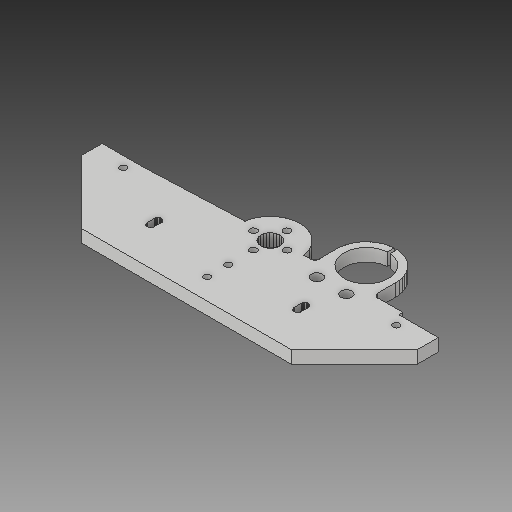
# Autodesk Inventor part: Rear-Bed-Holder-Lower
Saved by Autodesk Inventor 2017 (Build 210142000, 142)
## iProperties
Created: 2016-07-12
Part Number: Rear-Bed-Holder-Lower
Material: Generic
Document SubType Name: Modeling
Designer: joshmamo
Density: 1 g/cm^3
Appearance: Default
Author: joshmamo
Autodesk Inventor part; units mm, degrees
ref_plane "YZ Plane" through (0, 0, 0) normal (1, 0, 0) x (0, 1, 0)
ref_plane "XZ Plane" through (0, 0, 0) normal (0, 1, 0) x (-1, 0, 0)
ref_plane "XY Plane" through (0, 0, 0) normal (0, 0, 1) x (1, 0, 0)
sketch "Sketch1" plane through (0, 0, 0) normal (0, 1, 0) x (-1, 0, 0)
  line L0 (324.9839, 293.9621) -> (323.9081, 293.4902)
  line L1 (323.9081, 293.4902) -> (322.9911, 292.756)
  line L2 (322.9911, 292.756) -> (322.2953, 291.8095)
  line L3 (322.2953, 291.8095) -> (321.8683, 290.7151)
  line L4 (321.8683, 290.7151) -> (321.739, 289.5475)
  line L5 (321.739, 289.5475) -> (321.9163, 288.3862)
  line L6 (321.9163, 288.3862) -> (322.3882, 287.3104)
  line L7 (322.3882, 287.3104) -> (323.1224, 286.3934)
  line L8 (323.1224, 286.3934) -> (324.0689, 285.6977)
  line L9 (324.0689, 285.6977) -> (325.1633, 285.2706)
  line L10 (325.1633, 285.2706) -> (326.3309, 285.1413)
  line L11 (326.3309, 285.1413) -> (327.4922, 285.3187)
  line L12 (327.4922, 285.3187) -> (328.568, 285.7905)
  line L13 (328.568, 285.7905) -> (329.485, 286.5247)
  line L14 (329.485, 286.5247) -> (330.1807, 287.4713)
  line L15 (330.1807, 287.4713) -> (330.6078, 288.5656)
  line L16 (330.6078, 288.5656) -> (330.7371, 289.7332)
  line L17 (330.7371, 289.7332) -> (330.5598, 290.8945)
  line L18 (330.5598, 290.8945) -> (330.0879, 291.9703)
  line L19 (330.0879, 291.9703) -> (329.3537, 292.8873)
  line L20 (329.3537, 292.8873) -> (328.4072, 293.5831)
  line L21 (328.4072, 293.5831) -> (327.3128, 294.0101)
  line L22 (327.3128, 294.0101) -> (326.1452, 294.1394)
  line L23 (326.1452, 294.1394) -> (324.9839, 293.9621)
  line L24 (362.7103, 307.2904) -> (362.8801, 307.7004)
  line L25 (362.8801, 307.7004) -> (362.938, 308.1404)
  line L26 (362.938, 308.1404) -> (362.938, 311.5404)
  line L27 (362.938, 311.5404) -> (362.8801, 311.9804)
  line L28 (362.8801, 311.9804) -> (362.7103, 312.3904)
  line L29 (362.7103, 312.3904) -> (362.4401, 312.7425)
  line L30 (362.4401, 312.7425) -> (362.088, 313.0126)
  line L31 (362.088, 313.0126) -> (361.678, 313.1824)
  line L32 (361.678, 313.1824) -> (361.238, 313.2404)
  line L33 (361.238, 313.2404) -> (360.798, 313.1824)
  line L34 (360.798, 313.1824) -> (360.388, 313.0126)
  line L35 (360.388, 313.0126) -> (360.036, 312.7425)
  line L36 (360.036, 312.7425) -> (359.7658, 312.3904)
  line L37 (359.7658, 312.3904) -> (359.596, 311.9804)
  line L38 (359.596, 311.9804) -> (359.538, 311.5404)
  line L39 (359.538, 311.5404) -> (359.538, 308.1404)
  line L40 (359.538, 308.1404) -> (359.596, 307.7004)
  line L41 (359.596, 307.7004) -> (359.7658, 307.2904)
  line L42 (359.7658, 307.2904) -> (360.036, 306.9383)
  line L43 (360.036, 306.9383) -> (360.388, 306.6681)
  line L44 (360.388, 306.6681) -> (360.798, 306.4983)
  line L45 (360.798, 306.4983) -> (361.238, 306.4404)
  line L46 (361.238, 306.4404) -> (361.678, 306.4983)
  line L47 (361.678, 306.4983) -> (362.088, 306.6681)
  line L48 (362.088, 306.6681) -> (362.4401, 306.9383)
  line L49 (362.4401, 306.9383) -> (362.7103, 307.2904)
  line L50 (292.088, 306.6681) -> (292.4401, 306.9383)
  line L51 (292.4401, 306.9383) -> (292.7103, 307.2904)
  line L52 (292.7103, 307.2904) -> (292.8801, 307.7004)
  line L53 (292.8801, 307.7004) -> (292.938, 308.1404)
  line L54 (292.938, 308.1404) -> (292.938, 311.5404)
  line L55 (292.938, 311.5404) -> (292.8801, 311.9804)
  line L56 (292.8801, 311.9804) -> (292.7103, 312.3904)
  line L57 (292.7103, 312.3904) -> (292.4401, 312.7425)
  line L58 (292.4401, 312.7425) -> (292.088, 313.0126)
  line L59 (292.088, 313.0126) -> (291.678, 313.1824)
  line L60 (291.678, 313.1824) -> (291.238, 313.2404)
  line L61 (291.238, 313.2404) -> (290.798, 313.1824)
  line L62 (290.798, 313.1824) -> (290.388, 313.0126)
  line L63 (290.388, 313.0126) -> (290.036, 312.7425)
  line L64 (290.036, 312.7425) -> (289.7658, 312.3904)
  line L65 (289.7658, 312.3904) -> (289.596, 311.9804)
  line L66 (289.596, 311.9804) -> (289.538, 311.5404)
  line L67 (289.538, 311.5404) -> (289.538, 308.1404)
  line L68 (289.538, 308.1404) -> (289.596, 307.7004)
  line L69 (289.596, 307.7004) -> (289.7658, 307.2904)
  line L70 (289.7658, 307.2904) -> (290.036, 306.9383)
  line L71 (290.036, 306.9383) -> (290.388, 306.6681)
  line L72 (290.388, 306.6681) -> (290.798, 306.4983)
  line L73 (290.798, 306.4983) -> (291.238, 306.4404)
  line L74 (291.238, 306.4404) -> (291.678, 306.4983)
  line L75 (291.678, 306.4983) -> (292.088, 306.6681)
  line L76 (326.8705, 297.7695) -> (327.1965, 298.0306)
  line L77 (327.1965, 298.0306) -> (327.4439, 298.3671)
  line L78 (327.4439, 298.3671) -> (327.5957, 298.7562)
  line L79 (327.5957, 298.7562) -> (327.6417, 299.1714)
  line L80 (327.6417, 299.1714) -> (327.5786, 299.5843)
  line L81 (327.5786, 299.5843) -> (327.4109, 299.9668)
  line L82 (327.4109, 299.9668) -> (327.1498, 300.2928)
  line L83 (327.1498, 300.2928) -> (326.8133, 300.5402)
  line L84 (326.8133, 300.5402) -> (326.4242, 300.692)
  line L85 (326.4242, 300.692) -> (326.009, 300.738)
  line L86 (326.009, 300.738) -> (325.5961, 300.675)
  line L87 (325.5961, 300.675) -> (325.2136, 300.5072)
  line L88 (325.2136, 300.5072) -> (324.8876, 300.2461)
  line L89 (324.8876, 300.2461) -> (324.6402, 299.9096)
  line L90 (324.6402, 299.9096) -> (324.4883, 299.5205)
  line L91 (324.4883, 299.5205) -> (324.4424, 299.1053)
  line L92 (324.4424, 299.1053) -> (324.5054, 298.6924)
  line L93 (324.5054, 298.6924) -> (324.6732, 298.3099)
  line L94 (324.6732, 298.3099) -> (324.9342, 297.9839)
  line L95 (324.9342, 297.9839) -> (325.2708, 297.7365)
  line L96 (325.2708, 297.7365) -> (325.6599, 297.5847)
  line L97 (325.6599, 297.5847) -> (326.075, 297.5387)
  line L98 (326.075, 297.5387) -> (326.4879, 297.6017)
  line L99 (326.4879, 297.6017) -> (326.8705, 297.7695)
  line L100 (327.2625, 278.7736) -> (327.5885, 279.0346)
  line L101 (327.5885, 279.0346) -> (327.8359, 279.3712)
  line L102 (327.8359, 279.3712) -> (327.9877, 279.7603)
  line L103 (327.9877, 279.7603) -> (328.0337, 280.1754)
  line L104 (328.0337, 280.1754) -> (327.9707, 280.5883)
  line L105 (327.9707, 280.5883) -> (327.8029, 280.9708)
  line L106 (327.8029, 280.9708) -> (327.5418, 281.2969)
  line L107 (327.5418, 281.2969) -> (327.2053, 281.5442)
  line L108 (327.2053, 281.5442) -> (326.8162, 281.6961)
  line L109 (326.8162, 281.6961) -> (326.401, 281.7421)
  line L110 (326.401, 281.7421) -> (325.9881, 281.679)
  line L111 (325.9881, 281.679) -> (325.6056, 281.5112)
  line L112 (325.6056, 281.5112) -> (325.2796, 281.2502)
  line L113 (325.2796, 281.2502) -> (325.0322, 280.9136)
  line L114 (325.0322, 280.9136) -> (324.8804, 280.5245)
  line L115 (324.8804, 280.5245) -> (324.8344, 280.1094)
  line L116 (324.8344, 280.1094) -> (324.8974, 279.6965)
  line L117 (324.8974, 279.6965) -> (325.0652, 279.314)
  line L118 (325.0652, 279.314) -> (325.3263, 278.9879)
  line L119 (325.3263, 278.9879) -> (325.6628, 278.7405)
  line L120 (325.6628, 278.7405) -> (326.0519, 278.5887)
  line L121 (326.0519, 278.5887) -> (326.4671, 278.5427)
  line L122 (326.4671, 278.5427) -> (326.88, 278.6058)
  line L123 (326.88, 278.6058) -> (327.2625, 278.7736)
  line L124 (262.6237, 293.8404) -> (262.7835, 294.2263)
  line L125 (262.7835, 294.2263) -> (262.838, 294.6404)
  line L126 (262.838, 294.6404) -> (262.7835, 295.0545)
  line L127 (262.7835, 295.0545) -> (262.6237, 295.4404)
  line L128 (262.6237, 295.4404) -> (262.3694, 295.7717)
  line L129 (262.3694, 295.7717) -> (262.038, 296.026)
  line L130 (262.038, 296.026) -> (261.6522, 296.1859)
  line L131 (261.6522, 296.1859) -> (261.238, 296.2404)
  line L132 (261.238, 296.2404) -> (260.8239, 296.1859)
  line L133 (260.8239, 296.1859) -> (260.438, 296.026)
  line L134 (260.438, 296.026) -> (260.1067, 295.7717)
  line L135 (260.1067, 295.7717) -> (259.8524, 295.4404)
  line L136 (259.8524, 295.4404) -> (259.6926, 295.0545)
  line L137 (259.6926, 295.0545) -> (259.638, 294.6404)
  line L138 (259.638, 294.6404) -> (259.6926, 294.2263)
  line L139 (259.6926, 294.2263) -> (259.8524, 293.8404)
  line L140 (259.8524, 293.8404) -> (260.1067, 293.509)
  line L141 (260.1067, 293.509) -> (260.438, 293.2547)
  line L142 (260.438, 293.2547) -> (260.8239, 293.0949)
  line L143 (260.8239, 293.0949) -> (261.238, 293.0404)
  line L144 (261.238, 293.0404) -> (261.6522, 293.0949)
  line L145 (261.6522, 293.0949) -> (262.038, 293.2547)
  line L146 (262.038, 293.2547) -> (262.3694, 293.509)
  line L147 (262.3694, 293.509) -> (262.6237, 293.8404)
  line L148 (390.8239, 296.1859) -> (390.438, 296.026)
  line L149 (390.438, 296.026) -> (390.1067, 295.7717)
  line L150 (390.1067, 295.7717) -> (389.8524, 295.4404)
  line L151 (389.8524, 295.4404) -> (389.6926, 295.0545)
  line L152 (389.6926, 295.0545) -> (389.638, 294.6404)
  line L153 (389.638, 294.6404) -> (389.6926, 294.2263)
  line L154 (389.6926, 294.2263) -> (389.8524, 293.8404)
  line L155 (389.8524, 293.8404) -> (390.1067, 293.509)
  line L156 (390.1067, 293.509) -> (390.438, 293.2547)
  line L157 (390.438, 293.2547) -> (390.8239, 293.0949)
  line L158 (390.8239, 293.0949) -> (391.238, 293.0404)
  line L159 (391.238, 293.0404) -> (391.6522, 293.0949)
  line L160 (391.6522, 293.0949) -> (392.038, 293.2547)
  line L161 (392.038, 293.2547) -> (392.3694, 293.509)
  line L162 (392.3694, 293.509) -> (392.6237, 293.8404)
  line L163 (392.6237, 293.8404) -> (392.7835, 294.2263)
  line L164 (392.7835, 294.2263) -> (392.838, 294.6404)
  line L165 (392.838, 294.6404) -> (392.7835, 295.0545)
  line L166 (392.7835, 295.0545) -> (392.6237, 295.4404)
  line L167 (392.6237, 295.4404) -> (392.3694, 295.7717)
  line L168 (392.3694, 295.7717) -> (392.038, 296.026)
  line L169 (392.038, 296.026) -> (391.6522, 296.1859)
  line L170 (391.6522, 296.1859) -> (391.238, 296.2404)
  line L171 (391.238, 296.2404) -> (390.8239, 296.1859)
  line L172 (318.1419, 288.6731) -> (318.2938, 289.0622)
  line L173 (318.2938, 289.0622) -> (318.3397, 289.4774)
  line L174 (318.3397, 289.4774) -> (318.2767, 289.8903)
  line L175 (318.2767, 289.8903) -> (318.1089, 290.2728)
  line L176 (318.1089, 290.2728) -> (317.8479, 290.5988)
  line L177 (317.8479, 290.5988) -> (317.5113, 290.8462)
  line L178 (317.5113, 290.8462) -> (317.1222, 290.9981)
  line L179 (317.1222, 290.9981) -> (316.7071, 291.044)
  line L180 (316.7071, 291.044) -> (316.2942, 290.981)
  line L181 (316.2942, 290.981) -> (315.9116, 290.8132)
  line L182 (315.9116, 290.8132) -> (315.5856, 290.5521)
  line L183 (315.5856, 290.5521) -> (315.3382, 290.2156)
  line L184 (315.3382, 290.2156) -> (315.1864, 289.8265)
  line L185 (315.1864, 289.8265) -> (315.1404, 289.4114)
  line L186 (315.1404, 289.4114) -> (315.2035, 288.9985)
  line L187 (315.2035, 288.9985) -> (315.3712, 288.6159)
  line L188 (315.3712, 288.6159) -> (315.6323, 288.2899)
  line L189 (315.6323, 288.2899) -> (315.9688, 288.0425)
  line L190 (315.9688, 288.0425) -> (316.3579, 287.8907)
  line L191 (316.3579, 287.8907) -> (316.7731, 287.8447)
  line L192 (316.7731, 287.8447) -> (317.186, 287.9078)
  line L193 (317.186, 287.9078) -> (317.5685, 288.0755)
  line L194 (317.5685, 288.0755) -> (317.8945, 288.3366)
  line L195 (317.8945, 288.3366) -> (318.1419, 288.6731)
  line L196 (334.1994, 289.3905) -> (334.3672, 289.008)
  line L197 (334.3672, 289.008) -> (334.6282, 288.6819)
  line L198 (334.6282, 288.6819) -> (334.9648, 288.4345)
  line L199 (334.9648, 288.4345) -> (335.3539, 288.2827)
  line L200 (335.3539, 288.2827) -> (335.769, 288.2367)
  line L201 (335.769, 288.2367) -> (336.1819, 288.2998)
  line L202 (336.1819, 288.2998) -> (336.5644, 288.4675)
  line L203 (336.5644, 288.4675) -> (336.8905, 288.7286)
  line L204 (336.8905, 288.7286) -> (337.1379, 289.0651)
  line L205 (337.1379, 289.0651) -> (337.2897, 289.4542)
  line L206 (337.2897, 289.4542) -> (337.3357, 289.8694)
  line L207 (337.3357, 289.8694) -> (337.2726, 290.2823)
  line L208 (337.2726, 290.2823) -> (337.1049, 290.6648)
  line L209 (337.1049, 290.6648) -> (336.8438, 290.9908)
  line L210 (336.8438, 290.9908) -> (336.5073, 291.2382)
  line L211 (336.5073, 291.2382) -> (336.1182, 291.3901)
  line L212 (336.1182, 291.3901) -> (335.703, 291.436)
  line L213 (335.703, 291.436) -> (335.2901, 291.373)
  line L214 (335.2901, 291.373) -> (334.9076, 291.2052)
  line L215 (334.9076, 291.2052) -> (334.5815, 290.9442)
  line L216 (334.5815, 290.9442) -> (334.3342, 290.6076)
  line L217 (334.3342, 290.6076) -> (334.1823, 290.2185)
  line L218 (334.1823, 290.2185) -> (334.1364, 289.8034)
  line L219 (334.1364, 289.8034) -> (334.1994, 289.3905)
  line L220 (324.6214, 275.5909) -> (328.3127, 275.6512)
  line L221 (328.3127, 275.6512) -> (331.8627, 276.6649)
  line L222 (331.8627, 276.6649) -> (335.0293, 278.5628)
  line L223 (335.0293, 278.5628) -> (337.5969, 281.2156)
  line L224 (337.5969, 281.2156) -> (339.3903, 284.4425)
  line L225 (339.3903, 284.4425) -> (340.2064, 287.7002)
  line L226 (340.2064, 287.7002) -> (387.4849, 289.6404)
  line L227 (387.4849, 289.6404) -> (406.238, 289.6404)
  line L228 (406.238, 289.6404) -> (406.238, 299.6404)
  line L229 (406.238, 299.6404) -> (376.238, 329.6404)
  line L230 (376.238, 329.6404) -> (276.238, 329.6404)
  line L231 (276.238, 329.6404) -> (246.238, 299.6404)
  line L232 (246.238, 299.6404) -> (246.238, 289.6404)
  line L233 (246.238, 289.6404) -> (264.9912, 289.6404)
  line L234 (264.9912, 289.6404) -> (264.9912, 287.7002)
  line L235 (264.9912, 287.7002) -> (276.8912, 287.7002)
  line L236 (276.8912, 287.7002) -> (277.2559, 287.6683)
  line L237 (277.2559, 287.6683) -> (277.6094, 287.5736)
  line L238 (277.6094, 287.5736) -> (277.9412, 287.4189)
  line L239 (277.9412, 287.4189) -> (278.241, 287.2089)
  line L240 (278.241, 287.2089) -> (278.4999, 286.9501)
  line L241 (278.4999, 286.9501) -> (278.7098, 286.6502)
  line L242 (278.7098, 286.6502) -> (278.8645, 286.3185)
  line L243 (278.8645, 286.3185) -> (278.9593, 285.9649)
  line L244 (278.9593, 285.9649) -> (278.9912, 285.6002)
  line L245 (278.9912, 285.6002) -> (278.9912, 277.2002)
  line L246 (278.9912, 277.2002) -> (279.1035, 275.4307)
  line L247 (279.1035, 275.4307) -> (279.4385, 273.6896)
  line L248 (279.4385, 273.6896) -> (279.9909, 272.0048)
  line L249 (279.9909, 272.0048) -> (280.7518, 270.4034)
  line L250 (280.7518, 270.4034) -> (281.709, 268.9109)
  line L251 (281.709, 268.9109) -> (282.8472, 267.5514)
  line L252 (282.8472, 267.5514) -> (284.1481, 266.3467)
  line L253 (284.1481, 266.3467) -> (285.5909, 265.316)
  line L254 (285.5909, 265.316) -> (287.1523, 264.476)
  line L255 (287.1523, 264.476) -> (288.8073, 263.84)
  line L256 (288.8073, 263.84) -> (290.5295, 263.4184)
  line L257 (290.5295, 263.4184) -> (292.2912, 263.2177)
  line L258 (292.2912, 263.2177) -> (292.2912, 266.7236)
  line L259 (292.2912, 266.7236) -> (290.6547, 266.9635)
  line L260 (290.6547, 266.9635) -> (289.0762, 267.4574)
  line L261 (289.0762, 267.4574) -> (287.5948, 268.1931)
  line L262 (287.5948, 268.1931) -> (286.2473, 269.1522)
  line L263 (286.2473, 269.1522) -> (285.0672, 270.3111)
  line L264 (285.0672, 270.3111) -> (284.0837, 271.6409)
  line L265 (284.0837, 271.6409) -> (283.3212, 273.1086)
  line L266 (283.3212, 273.1086) -> (282.7986, 274.6779)
  line L267 (282.7986, 274.6779) -> (282.529, 276.3098)
  line L268 (282.529, 276.3098) -> (282.519, 277.9637)
  line L269 (282.519, 277.9637) -> (282.7688, 279.5988)
  line L270 (282.7688, 279.5988) -> (283.2723, 281.1743)
  line L271 (283.2723, 281.1743) -> (284.0169, 282.6511)
  line L272 (284.0169, 282.6511) -> (284.9842, 283.9928)
  line L273 (284.9842, 283.9928) -> (286.1502, 285.1659)
  line L274 (286.1502, 285.1659) -> (287.486, 286.1413)
  line L275 (287.486, 286.1413) -> (288.9583, 286.8949)
  line L276 (288.9583, 286.8949) -> (290.5307, 287.4079)
  line L277 (290.5307, 287.4079) -> (292.1642, 287.6676)
  line L278 (292.1642, 287.6676) -> (293.8182, 287.6676)
  line L279 (293.8182, 287.6676) -> (295.4517, 287.4079)
  line L280 (295.4517, 287.4079) -> (297.0241, 286.8949)
  line L281 (297.0241, 286.8949) -> (298.4964, 286.1413)
  line L282 (298.4964, 286.1413) -> (299.8322, 285.1659)
  line L283 (299.8322, 285.1659) -> (300.9982, 283.9928)
  line L284 (300.9982, 283.9928) -> (301.9655, 282.6511)
  line L285 (301.9655, 282.6511) -> (302.7101, 281.1743)
  line L286 (302.7101, 281.1743) -> (303.2136, 279.5988)
  line L287 (303.2136, 279.5988) -> (303.4634, 277.9637)
  line L288 (303.4634, 277.9637) -> (303.4534, 276.3098)
  line L289 (303.4534, 276.3098) -> (303.1837, 274.6779)
  line L290 (303.1837, 274.6779) -> (302.6612, 273.1086)
  line L291 (302.6612, 273.1086) -> (301.8987, 271.6409)
  line L292 (301.8987, 271.6409) -> (300.9152, 270.3111)
  line L293 (300.9152, 270.3111) -> (299.7351, 269.1522)
  line L294 (299.7351, 269.1522) -> (298.3876, 268.1931)
  line L295 (298.3876, 268.1931) -> (296.9062, 267.4574)
  line L296 (296.9062, 267.4574) -> (295.3277, 266.9635)
  line L297 (295.3277, 266.9635) -> (293.6912, 266.7236)
  line L298 (293.6912, 266.7236) -> (293.6912, 263.2177)
  line L299 (293.6912, 263.2177) -> (295.4529, 263.4184)
  line L300 (295.4529, 263.4184) -> (297.175, 263.84)
  line L301 (297.175, 263.84) -> (298.8301, 264.476)
  line L302 (298.8301, 264.476) -> (300.3915, 265.316)
  line L303 (300.3915, 265.316) -> (301.8343, 266.3467)
  line L304 (301.8343, 266.3467) -> (303.1352, 267.5514)
  line L305 (303.1352, 267.5514) -> (304.2733, 268.9109)
  line L306 (304.2733, 268.9109) -> (305.2306, 270.4034)
  line L307 (305.2306, 270.4034) -> (305.9915, 272.0048)
  line L308 (305.9915, 272.0048) -> (306.5439, 273.6896)
  line L309 (306.5439, 273.6896) -> (306.8789, 275.4307)
  line L310 (306.8789, 275.4307) -> (306.9912, 277.2002)
  line L311 (306.9912, 277.2002) -> (306.9912, 285.6002)
  line L312 (306.9912, 285.6002) -> (307.0231, 285.9649)
  line L313 (307.0231, 285.9649) -> (307.1178, 286.3185)
  line L314 (307.1178, 286.3185) -> (307.2725, 286.6502)
  line L315 (307.2725, 286.6502) -> (307.4825, 286.9501)
  line L316 (307.4825, 286.9501) -> (307.7413, 287.2089)
  line L317 (307.7413, 287.2089) -> (308.0412, 287.4189)
  line L318 (308.0412, 287.4189) -> (308.373, 287.5736)
  line L319 (308.373, 287.5736) -> (308.7265, 287.6683)
  line L320 (308.7265, 287.6683) -> (309.0912, 287.7002)
  line L321 (309.0912, 287.7002) -> (312.2467, 287.7002)
  line L322 (312.2467, 287.7002) -> (312.2489, 287.5657)
  line L323 (312.2489, 287.5657) -> (313.2626, 284.0157)
  line L324 (313.2626, 284.0157) -> (315.1604, 280.8491)
  line L325 (315.1604, 280.8491) -> (317.8133, 278.2815)
  line L326 (317.8133, 278.2815) -> (321.0402, 276.4881)
  line L327 (321.0402, 276.4881) -> (324.6214, 275.5909)
  line L328 (376.238, 329.6404) -> (276.238, 329.6404)
  line L329 (276.238, 329.6404) -> (246.238, 299.6404)
  line L330 (246.238, 299.6404) -> (246.238, 289.6404)
  line L331 (246.238, 289.6404) -> (264.9912, 289.6404)
  line L332 (264.9912, 289.6404) -> (264.9912, 287.7002)
  line L333 (264.9912, 287.7002) -> (276.8912, 287.7002)
  line L334 (276.8912, 287.7002) -> (277.2559, 287.6683)
  line L335 (277.2559, 287.6683) -> (277.6094, 287.5736)
  line L336 (277.6094, 287.5736) -> (277.9412, 287.4189)
  line L337 (277.9412, 287.4189) -> (278.241, 287.2089)
  line L338 (278.241, 287.2089) -> (278.4999, 286.9501)
  line L339 (278.4999, 286.9501) -> (278.7098, 286.6502)
  line L340 (278.7098, 286.6502) -> (278.8645, 286.3185)
  line L341 (278.8645, 286.3185) -> (278.9593, 285.9649)
  line L342 (278.9593, 285.9649) -> (278.9912, 285.6002)
  line L343 (278.9912, 285.6002) -> (278.9912, 277.2002)
  line L344 (278.9912, 277.2002) -> (279.1035, 275.4307)
  line L345 (279.1035, 275.4307) -> (279.4385, 273.6896)
  line L346 (279.4385, 273.6896) -> (279.9909, 272.0048)
  line L347 (279.9909, 272.0048) -> (280.7518, 270.4034)
  line L348 (280.7518, 270.4034) -> (281.709, 268.9109)
  line L349 (281.709, 268.9109) -> (282.8472, 267.5514)
  line L350 (282.8472, 267.5514) -> (284.1481, 266.3467)
  line L351 (284.1481, 266.3467) -> (285.5909, 265.316)
  line L352 (285.5909, 265.316) -> (287.1523, 264.476)
  line L353 (287.1523, 264.476) -> (288.8073, 263.84)
  line L354 (288.8073, 263.84) -> (290.5295, 263.4184)
  line L355 (290.5295, 263.4184) -> (292.2912, 263.2177)
  line L356 (292.2912, 263.2177) -> (292.2912, 266.7236)
  line L357 (292.2912, 266.7236) -> (290.6547, 266.9635)
  line L358 (290.6547, 266.9635) -> (289.0762, 267.4574)
  line L359 (289.0762, 267.4574) -> (287.5948, 268.1931)
  line L360 (287.5948, 268.1931) -> (286.2473, 269.1522)
  line L361 (286.2473, 269.1522) -> (285.0672, 270.3111)
  line L362 (285.0672, 270.3111) -> (284.0837, 271.6409)
  line L363 (284.0837, 271.6409) -> (283.3212, 273.1086)
  line L364 (283.3212, 273.1086) -> (282.7986, 274.6779)
  line L365 (282.7986, 274.6779) -> (282.529, 276.3098)
  line L366 (282.529, 276.3098) -> (282.519, 277.9637)
  line L367 (282.519, 277.9637) -> (282.7688, 279.5988)
  line L368 (282.7688, 279.5988) -> (283.2723, 281.1743)
  line L369 (283.2723, 281.1743) -> (284.0169, 282.6511)
  line L370 (284.0169, 282.6511) -> (284.9842, 283.9928)
  line L371 (284.9842, 283.9928) -> (286.1502, 285.1659)
  line L372 (286.1502, 285.1659) -> (287.486, 286.1413)
  line L373 (287.486, 286.1413) -> (288.9583, 286.8949)
  line L374 (288.9583, 286.8949) -> (290.5307, 287.4079)
  line L375 (290.5307, 287.4079) -> (292.1642, 287.6676)
  line L376 (292.1642, 287.6676) -> (293.8182, 287.6676)
  line L377 (293.8182, 287.6676) -> (295.4517, 287.4079)
  line L378 (295.4517, 287.4079) -> (297.0241, 286.8949)
  line L379 (297.0241, 286.8949) -> (298.4964, 286.1413)
  line L380 (298.4964, 286.1413) -> (299.8322, 285.1659)
  line L381 (299.8322, 285.1659) -> (300.9982, 283.9928)
  line L382 (300.9982, 283.9928) -> (301.9655, 282.6511)
  line L383 (301.9655, 282.6511) -> (302.7101, 281.1743)
  line L384 (302.7101, 281.1743) -> (303.2136, 279.5988)
  line L385 (303.2136, 279.5988) -> (303.4634, 277.9637)
  line L386 (303.4634, 277.9637) -> (303.4534, 276.3098)
  line L387 (303.4534, 276.3098) -> (303.1837, 274.6779)
  line L388 (303.1837, 274.6779) -> (302.6612, 273.1086)
  line L389 (302.6612, 273.1086) -> (301.8987, 271.6409)
  line L390 (301.8987, 271.6409) -> (300.9152, 270.3111)
  line L391 (300.9152, 270.3111) -> (299.7351, 269.1522)
  line L392 (299.7351, 269.1522) -> (298.3876, 268.1931)
  line L393 (298.3876, 268.1931) -> (296.9062, 267.4574)
  line L394 (296.9062, 267.4574) -> (295.3277, 266.9635)
  line L395 (295.3277, 266.9635) -> (293.6912, 266.7236)
  line L396 (293.6912, 266.7236) -> (293.6912, 263.2177)
  line L397 (293.6912, 263.2177) -> (295.4529, 263.4184)
  line L398 (295.4529, 263.4184) -> (297.175, 263.84)
  line L399 (297.175, 263.84) -> (298.8301, 264.476)
  line L400 (298.8301, 264.476) -> (300.3915, 265.316)
  line L401 (300.3915, 265.316) -> (301.8343, 266.3467)
  line L402 (301.8343, 266.3467) -> (303.1352, 267.5514)
  line L403 (303.1352, 267.5514) -> (304.2733, 268.9109)
  line L404 (304.2733, 268.9109) -> (305.2306, 270.4034)
  line L405 (305.2306, 270.4034) -> (305.9915, 272.0048)
  line L406 (305.9915, 272.0048) -> (306.5439, 273.6896)
  line L407 (306.5439, 273.6896) -> (306.8789, 275.4307)
  line L408 (306.8789, 275.4307) -> (306.9912, 277.2002)
  line L409 (306.9912, 277.2002) -> (306.9912, 285.6002)
  line L410 (306.9912, 285.6002) -> (307.0231, 285.9649)
  line L411 (307.0231, 285.9649) -> (307.1178, 286.3185)
  line L412 (307.1178, 286.3185) -> (307.2725, 286.6502)
  line L413 (307.2725, 286.6502) -> (307.4825, 286.9501)
  line L414 (307.4825, 286.9501) -> (307.7413, 287.2089)
  line L415 (307.7413, 287.2089) -> (308.0412, 287.4189)
  line L416 (308.0412, 287.4189) -> (308.373, 287.5736)
  line L417 (308.373, 287.5736) -> (308.7265, 287.6683)
  line L418 (308.7265, 287.6683) -> (309.0912, 287.7002)
  line L419 (309.0912, 287.7002) -> (312.2467, 287.7002)
  line L420 (312.2467, 287.7002) -> (312.2489, 287.5657)
  line L421 (312.2489, 287.5657) -> (313.2626, 284.0157)
  line L422 (313.2626, 284.0157) -> (315.1604, 280.8491)
  line L423 (315.1604, 280.8491) -> (317.8133, 278.2815)
  line L424 (317.8133, 278.2815) -> (321.0402, 276.4881)
  line L425 (321.0402, 276.4881) -> (324.6214, 275.5909)
  line L426 (324.6214, 275.5909) -> (328.3127, 275.6512)
  line L427 (328.3127, 275.6512) -> (331.8627, 276.6649)
  line L428 (331.8627, 276.6649) -> (335.0293, 278.5628)
  line L429 (335.0293, 278.5628) -> (337.5969, 281.2156)
  line L430 (337.5969, 281.2156) -> (339.3903, 284.4425)
  line L431 (339.3903, 284.4425) -> (340.2064, 287.7002)
  line L432 (340.2064, 287.7002) -> (387.4849, 289.6404)
  line L433 (387.4849, 289.6404) -> (406.238, 289.6404)
  line L434 (406.238, 289.6404) -> (406.238, 299.6404)
  line L435 (406.238, 299.6404) -> (376.238, 329.6404)
  line L436 (376.238, 329.6404) -> (406.238, 299.6404)
  line L437 (406.238, 299.6404) -> (406.238, 289.6404)
  line L438 (406.238, 289.6404) -> (387.4849, 289.6404)
  line L439 (387.4849, 289.6404) -> (340.2064, 287.7002)
  line L440 (340.2064, 287.7002) -> (339.3903, 284.4425)
  line L441 (339.3903, 284.4425) -> (337.5969, 281.2156)
  line L442 (337.5969, 281.2156) -> (335.0293, 278.5628)
  line L443 (335.0293, 278.5628) -> (331.8627, 276.6649)
  line L444 (331.8627, 276.6649) -> (328.3127, 275.6512)
  line L445 (328.3127, 275.6512) -> (324.6214, 275.5909)
  line L446 (324.6214, 275.5909) -> (321.0402, 276.4881)
  line L447 (321.0402, 276.4881) -> (317.8133, 278.2815)
  line L448 (317.8133, 278.2815) -> (315.1604, 280.8491)
  line L449 (315.1604, 280.8491) -> (313.2626, 284.0157)
  line L450 (313.2626, 284.0157) -> (312.2489, 287.5657)
  line L451 (312.2489, 287.5657) -> (312.2467, 287.7002)
  line L452 (312.2467, 287.7002) -> (309.0912, 287.7002)
  line L453 (309.0912, 287.7002) -> (308.7265, 287.6683)
  line L454 (308.7265, 287.6683) -> (308.373, 287.5736)
  line L455 (308.373, 287.5736) -> (308.0412, 287.4189)
  line L456 (308.0412, 287.4189) -> (307.7413, 287.2089)
  line L457 (307.7413, 287.2089) -> (307.4825, 286.9501)
  line L458 (307.4825, 286.9501) -> (307.2725, 286.6502)
  line L459 (307.2725, 286.6502) -> (307.1178, 286.3185)
  line L460 (307.1178, 286.3185) -> (307.0231, 285.9649)
  line L461 (307.0231, 285.9649) -> (306.9912, 285.6002)
  line L462 (306.9912, 285.6002) -> (306.9912, 277.2002)
  line L463 (306.9912, 277.2002) -> (306.8789, 275.4307)
  line L464 (306.8789, 275.4307) -> (306.5439, 273.6896)
  line L465 (306.5439, 273.6896) -> (305.9915, 272.0048)
  line L466 (305.9915, 272.0048) -> (305.2306, 270.4034)
  line L467 (305.2306, 270.4034) -> (304.2733, 268.9109)
  line L468 (304.2733, 268.9109) -> (303.1352, 267.5514)
  line L469 (303.1352, 267.5514) -> (301.8343, 266.3467)
  line L470 (301.8343, 266.3467) -> (300.3915, 265.316)
  line L471 (300.3915, 265.316) -> (298.8301, 264.476)
  line L472 (298.8301, 264.476) -> (297.175, 263.84)
  line L473 (297.175, 263.84) -> (295.4529, 263.4184)
  line L474 (295.4529, 263.4184) -> (293.6912, 263.2177)
  line L475 (293.6912, 263.2177) -> (293.6912, 266.7236)
  line L476 (293.6912, 266.7236) -> (295.3277, 266.9635)
  line L477 (295.3277, 266.9635) -> (296.9062, 267.4574)
  line L478 (296.9062, 267.4574) -> (298.3876, 268.1931)
  line L479 (298.3876, 268.1931) -> (299.7351, 269.1522)
  line L480 (299.7351, 269.1522) -> (300.9152, 270.3111)
  line L481 (300.9152, 270.3111) -> (301.8987, 271.6409)
  line L482 (301.8987, 271.6409) -> (302.6612, 273.1086)
  line L483 (302.6612, 273.1086) -> (303.1837, 274.6779)
  line L484 (303.1837, 274.6779) -> (303.4534, 276.3098)
  line L485 (303.4534, 276.3098) -> (303.4634, 277.9637)
  line L486 (303.4634, 277.9637) -> (303.2136, 279.5988)
  line L487 (303.2136, 279.5988) -> (302.7101, 281.1743)
  line L488 (302.7101, 281.1743) -> (301.9655, 282.6511)
  line L489 (301.9655, 282.6511) -> (300.9982, 283.9928)
  line L490 (300.9982, 283.9928) -> (299.8322, 285.1659)
  line L491 (299.8322, 285.1659) -> (298.4964, 286.1413)
  line L492 (298.4964, 286.1413) -> (297.0241, 286.8949)
  line L493 (297.0241, 286.8949) -> (295.4517, 287.4079)
  line L494 (295.4517, 287.4079) -> (293.8182, 287.6676)
  line L495 (293.8182, 287.6676) -> (292.1642, 287.6676)
  line L496 (292.1642, 287.6676) -> (290.5307, 287.4079)
  line L497 (290.5307, 287.4079) -> (288.9583, 286.8949)
  line L498 (288.9583, 286.8949) -> (287.486, 286.1413)
  line L499 (287.486, 286.1413) -> (286.1502, 285.1659)
  line L500 (286.1502, 285.1659) -> (284.9842, 283.9928)
  line L501 (284.9842, 283.9928) -> (284.0169, 282.6511)
  line L502 (284.0169, 282.6511) -> (283.2723, 281.1743)
  line L503 (283.2723, 281.1743) -> (282.7688, 279.5988)
  line L504 (282.7688, 279.5988) -> (282.519, 277.9637)
  line L505 (282.519, 277.9637) -> (282.529, 276.3098)
  line L506 (282.529, 276.3098) -> (282.7986, 274.6779)
  line L507 (282.7986, 274.6779) -> (283.3212, 273.1086)
  line L508 (283.3212, 273.1086) -> (284.0837, 271.6409)
  line L509 (284.0837, 271.6409) -> (285.0672, 270.3111)
  line L510 (285.0672, 270.3111) -> (286.2473, 269.1522)
  line L511 (286.2473, 269.1522) -> (287.5948, 268.1931)
  line L512 (287.5948, 268.1931) -> (289.0762, 267.4574)
  line L513 (289.0762, 267.4574) -> (290.6547, 266.9635)
  line L514 (290.6547, 266.9635) -> (292.2912, 266.7236)
  line L515 (292.2912, 266.7236) -> (292.2912, 263.2177)
  line L516 (292.2912, 263.2177) -> (290.5295, 263.4184)
  line L517 (290.5295, 263.4184) -> (288.8073, 263.84)
  line L518 (288.8073, 263.84) -> (287.1523, 264.476)
  line L519 (287.1523, 264.476) -> (285.5909, 265.316)
  line L520 (285.5909, 265.316) -> (284.1481, 266.3467)
  line L521 (284.1481, 266.3467) -> (282.8472, 267.5514)
  line L522 (282.8472, 267.5514) -> (281.709, 268.9109)
  line L523 (281.709, 268.9109) -> (280.7518, 270.4034)
  line L524 (280.7518, 270.4034) -> (279.9909, 272.0048)
  line L525 (279.9909, 272.0048) -> (279.4385, 273.6896)
  line L526 (279.4385, 273.6896) -> (279.1035, 275.4307)
  line L527 (279.1035, 275.4307) -> (278.9912, 277.2002)
  line L528 (278.9912, 277.2002) -> (278.9912, 285.6002)
  line L529 (278.9912, 285.6002) -> (278.9593, 285.9649)
  line L530 (278.9593, 285.9649) -> (278.8645, 286.3185)
  line L531 (278.8645, 286.3185) -> (278.7098, 286.6502)
  line L532 (278.7098, 286.6502) -> (278.4999, 286.9501)
  line L533 (278.4999, 286.9501) -> (278.241, 287.2089)
  line L534 (278.241, 287.2089) -> (277.9412, 287.4189)
  line L535 (277.9412, 287.4189) -> (277.6094, 287.5736)
  line L536 (277.6094, 287.5736) -> (277.2559, 287.6683)
  line L537 (277.2559, 287.6683) -> (276.8912, 287.7002)
  line L538 (276.8912, 287.7002) -> (264.9912, 287.7002)
  line L539 (264.9912, 287.7002) -> (264.9912, 289.6404)
  line L540 (264.9912, 289.6404) -> (246.238, 289.6404)
  line L541 (246.238, 289.6404) -> (246.238, 299.6404)
  line L542 (246.238, 299.6404) -> (276.238, 329.6404)
  circle A0 centre (326.238, 319.6404) radius 1.6
  circle A1 centre (326.238, 309.6404) radius 1.6
  line L543 (326.238, 329.6404) -> (336.238, 329.6404)
  circle A2 centre (285.9912, 293.6676) radius 2.6
  circle A3 centre (299.9912, 293.6676) radius 2.6
  point P0 (0, 0)
  constraints: 1088 end point, 4 centre point
extrude "Extrusion1" add sketch "Sketch1" along normal blind 6
sketch "Sketch2" plane through (0, 6, 0) normal (0, 1, 0) x (1, 0, 0)
  line L0 (-259.638, -294.6404) -> (-259.6926, -295.0545) projected
  line L1 (-262.838, -294.6404) -> (-259.638, -294.6404)
  circle A0 centre (-285.9912, -293.6676) radius 2.6 projected
  circle A1 centre (-299.9912, -293.6676) radius 2.6 projected
  line L2 (-318.3397, -289.4774) -> (-318.2938, -289.0622) projected
  line L3 (-315.1404, -289.4114) -> (-315.1864, -289.8265) projected
  line L4 (-318.3397, -289.4774) -> (-315.1404, -289.4114)
  line L5 (-328.0337, -280.1754) -> (-327.9877, -279.7603) projected
  line L6 (-324.8974, -279.6965) -> (-324.8344, -280.1094) projected
  line L7 (-328.0337, -280.1754) -> (-324.8344, -280.1094)
  line L8 (-327.6417, -299.1714) -> (-327.5957, -298.7562) projected
  line L9 (-324.4424, -299.1053) -> (-324.5054, -298.6924) projected
  line L10 (-327.6417, -299.1714) -> (-324.4424, -299.1053)
  line L11 (-330.7371, -289.7332) -> (-330.6078, -288.5656) projected
  line L12 (-321.739, -289.5475) -> (-321.9163, -288.3862) projected
  line L13 (-330.7371, -289.7332) -> (-321.739, -289.5475)
  line L14 (-337.3357, -289.8694) -> (-337.2897, -289.4542) projected
  line L15 (-334.1364, -289.8034) -> (-334.1994, -289.3905) projected
  line L16 (-337.3357, -289.8694) -> (-334.1364, -289.8034)
  circle A2 centre (-326.238, -309.6404) radius 1.6 projected
  circle A3 centre (-326.238, -319.6404) radius 1.6 projected
  line L17 (-392.838, -294.6404) -> (-389.638, -294.6404)
  line L18 (-303.4634, -277.9637) -> (-303.4534, -276.3098) projected
  line L19 (-303.4584, -277.1368) -> (-282.524, -277.1368)
  line L20 (-282.529, -276.3098) -> (-282.519, -277.9637) projected
  point P0 (0, 0)
  point P1 (-261.238, -294.6404)
  point P2 (-292.9912, -277.1368)
  point P3 (-316.7401, -289.4444)
  point P4 (-326.238, -289.6404)
  point P5 (-326.434, -280.1424)
  point P6 (-326.042, -299.1383)
  point P7 (-335.736, -289.8364)
  point P8 (-391.238, -294.6404)
  constraints: 16 end point, 10 midpoint, 4 coincident, 2 horizontal
hole "Hole1" at (-261.238, 6, 294.6404) at (-316.7401, 6, 289.4444) at (-326.434, 6, 280.1424) at (-326.042, 6, 299.1383) at (-335.736, 6, 289.8364) at (-326.238, 6, 309.6404) at (-326.238, 6, 319.6404) at (-391.238, 6, 294.6404) direction (0, -1, 0) diameter 3.2 depth 8 tip angle 118
sketch "Sketch3" plane through (0, 6, 0) normal (0, 1, 0) x (1, 0, 0)
  line L0 (-282.529, -276.3098) -> (-282.519, -277.9637) projected
  line L1 (-303.4634, -277.9637) -> (-303.4534, -276.3098) projected
  line L2 (-282.529, -276.3098) -> (-282.519, -277.9637) projected
  line L3 (-282.524, -277.1368) -> (-303.4584, -277.1368)
  point P0 (0, 0)
  point P1 (-292.9912, -277.1368)
  constraints: 3 midpoint, 2 end point
hole "Hole2" at (-292.9912, 6, 277.1368) direction (0, -1, 0) diameter 21.2 depth 8 tip angle 118
sketch "Sketch4" plane through (0, 0, 0) normal (0, -1, 0) x (1, 0, 0)
  line L0 (-317.6003, 282.57) -> (-313.1587, 288.6908)
  line L1 (-313.1587, 288.6908) -> (-313.6057, 295.8984)
  line L2 (-313.6057, 295.8984) -> (-329.0825, 303.2736)
  line L3 (-329.0825, 303.2736) -> (-339.5307, 292.2946)
  line L4 (-339.5307, 292.2946) -> (-338.1266, 284.2947)
  line L5 (-338.1266, 284.2947) -> (-327.2387, 276.9016)
  line L6 (-327.2387, 276.9016) -> (-320.3814, 278.1052)
  line L7 (-320.3814, 278.1052) -> (-320.3814, 281.6796)
  line L8 (-320.3814, 281.6796) -> (-327.6298, 283.8298)
  line L9 (-327.6298, 283.8298) -> (-331.917, 285.8728)
  line L10 (-331.917, 285.8728) -> (-332.3152, 292.2946)
  line L11 (-332.3152, 292.2946) -> (-330.3754, 296.3652)
  line L12 (-330.3754, 296.3652) -> (-324.1012, 296.7543)
  line L13 (-324.1012, 296.7543) -> (-319.5841, 290.5905)
  line L14 (-319.5841, 290.5905) -> (-318.782, 283.1331)
  line L15 (-318.782, 283.1331) -> (-317.6003, 282.57)
  point P0 (0, 0)
  constraints: 32 end point, 4 perpendicular, 2 parallel, 1 vertical
extrude "Extrusion2" add sketch "Sketch4" against normal blind 6
sketch "Sketch5" plane through (0, 0, 0) normal (0, -1, 0) x (1, 0, 0)
  circle A0 centre (-326.2243, 281.6404) radius 1.7 projected
  circle A1 centre (-318.2569, 289.6728) radius 1.7 projected
  circle A2 centre (-326.2894, 297.6402) radius 1.7 projected
  circle A3 centre (-334.2568, 289.6077) radius 1.7 projected
  point P0 (0, 0)
extrude "Extrusion3" cut sketch "Sketch5" against normal blind 6
body "Solid1"
